Autodesk Fusion 360 part; units mm, degrees
(part 3 of 11)
  spline S32 degree 5 poles (-12.9257, -25.5744) (-12.9262, -25.5771) (-12.9273, -25.5825) (-12.9286, -25.5906) (-12.93, -25.6015) (-12.9313, -25.6152) (-12.9322, -25.629) (-12.9328, -25.6428) (-12.9334, -25.6566) (-12.9338, -25.6705) (-12.9341, -25.6844) (-12.9343, -25.6983) (-12.9344, -25.7122) (-12.9342, -25.7262) (-12.9339, -25.7401) (-12.9334, -25.7542) (-12.9328, -25.7682) (-12.932, -25.7822) (-12.9311, -25.7963) (-12.9302, -25.8104) (-12.9291, -25.8245) (-12.9279, -25.8386) (-12.9266, -25.8527) (-12.9252, -25.8669) (-12.9236, -25.8811) (-12.922, -25.8952) (-12.9202, -25.9094) (-12.9184, -25.9236) (-12.9164, -25.9378) (-12.9144, -25.9521) (-12.9122, -25.9663) (-12.91, -25.9805) (-12.9077, -25.9948) (-12.9052, -26.0091) (-12.9027, -26.0233) (-12.9001, -26.0376) (-12.8974, -26.0519) (-12.8946, -26.0662) (-12.8917, -26.0805) (-12.8887, -26.0948) (-12.8856, -26.1091) (-12.8825, -26.1235) (-12.8792, -26.1378) (-12.8759, -26.1521) (-12.8725, -26.1665) (-12.869, -26.1808) (-12.8655, -26.1952) (-12.8618, -26.2096) (-12.8581, -26.2239) (-12.8542, -26.2383) (-12.8503, -26.2527) (-12.8464, -26.267) (-12.8423, -26.2814) (-12.8382, -26.2958) (-12.834, -26.3102) (-12.8297, -26.3246) (-12.8253, -26.339) (-12.8209, -26.3534) (-12.8163, -26.3678) (-12.8117, -26.3822) (-12.8071, -26.3966) (-12.8023, -26.4109) (-12.7975, -26.4253) (-12.7926, -26.4397) (-12.7876, -26.4541) (-12.7826, -26.4685) (-12.7774, -26.4829) (-12.7722, -26.4973) (-12.767, -26.5117) (-12.7616, -26.5261) (-12.7562, -26.5405) (-12.7518, -26.5521) (-12.7485, -26.5607) (-12.7463, -26.5664) (-12.7452, -26.5693) knots 0 0 0 0 0 0 0.01428571 0.02857143 0.04285714 0.05714286 0.07142857 0.08571429 0.1 0.11428571 0.12857143 0.14285714 0.15714286 0.17142857 0.18571429 0.2 0.21428571 0.22857143 0.24285714 0.25714286 0.27142857 0.28571429 0.3 0.31428571 0.32857143 0.34285714 0.35714286 0.37142857 0.38571429 0.4 0.41428571 0.42857143 0.44285714 0.45714286 0.47142857 0.48571429 0.5 0.51428571 0.52857143 0.54285714 0.55714286 0.57142857 0.58571429 0.6 0.61428571 0.62857143 0.64285714 0.65714286 0.67142857 0.68571429 0.7 0.71428571 0.72857143 0.74285714 0.75714286 0.77142857 0.78571429 0.8 0.81428571 0.82857143 0.84285714 0.85714286 0.87142857 0.88571429 0.9 0.91428571 0.92857143 0.94285714 0.95714286 0.97142857 0.98571429 1 1 1 1 1 1
  arc A66 (-12.7452, -26.5693) -> (-12.3546, -26.6175) centre (-11.6741, -19.5) ccw
  spline S33 degree 5 poles (-12.3546, -26.6175) (-12.3528, -26.615) (-12.3493, -26.61) (-12.344, -26.6024) (-12.3369, -26.5923) (-12.3282, -26.5797) (-12.3195, -26.567) (-12.3109, -26.5543) (-12.3023, -26.5416) (-12.2939, -26.5289) (-12.2855, -26.5161) (-12.2771, -26.5034) (-12.2689, -26.4906) (-12.2607, -26.4778) (-12.2526, -26.465) (-12.2446, -26.4522) (-12.2366, -26.4393) (-12.2287, -26.4265) (-12.2209, -26.4136) (-12.2131, -26.4007) (-12.2055, -26.3878) (-12.1979, -26.3749) (-12.1904, -26.3619) (-12.183, -26.3489) (-12.1756, -26.336) (-12.1683, -26.323) (-12.1611, -26.31) (-12.154, -26.2969) (-12.147, -26.2839) (-12.14, -26.2708) (-12.1331, -26.2578) (-12.1263, -26.2447) (-12.1196, -26.2316) (-12.113, -26.2185) (-12.1065, -26.2053) (-12.1, -26.1922) (-12.0936, -26.179) (-12.0874, -26.1659) (-12.0812, -26.1527) (-12.0751, -26.1395) (-12.069, -26.1263) (-12.0631, -26.113) (-12.0573, -26.0998) (-12.0516, -26.0865) (-12.0459, -26.0733) (-12.0404, -26.06) (-12.0349, -26.0467) (-12.0296, -26.0334) (-12.0243, -26.02) (-12.0192, -26.0067) (-12.0141, -25.9933) (-12.0092, -25.98) (-12.0044, -25.9666) (-11.9997, -25.9532) (-11.9951, -25.9398) (-11.9906, -25.9264) (-11.9862, -25.913) (-11.982, -25.8995) (-11.9778, -25.8861) (-11.9738, -25.8726) (-11.9699, -25.8592) (-11.9662, -25.8457) (-11.9627, -25.8322) (-11.9593, -25.8186) (-11.9561, -25.8051) (-11.9531, -25.7916) (-11.9501, -25.778) (-11.9472, -25.7645) (-11.9445, -25.7509) (-11.942, -25.7373) (-11.9399, -25.7237) (-11.9387, -25.7128) (-11.938, -25.7046) (-11.9377, -25.6991) (-11.9376, -25.6964) knots -1 -1 -1 -1 -1 -1 -0.98571429 -0.97142857 -0.95714286 -0.94285714 -0.92857143 -0.91428571 -0.9 -0.88571429 -0.87142857 -0.85714286 -0.84285714 -0.82857143 -0.81428571 -0.8 -0.78571429 -0.77142857 -0.75714286 -0.74285714 -0.72857143 -0.71428571 -0.7 -0.68571429 -0.67142857 -0.65714286 -0.64285714 -0.62857143 -0.61428571 -0.6 -0.58571429 -0.57142857 -0.55714286 -0.54285714 -0.52857143 -0.51428571 -0.5 -0.48571429 -0.47142857 -0.45714286 -0.44285714 -0.42857143 -0.41428571 -0.4 -0.38571429 -0.37142857 -0.35714286 -0.34285714 -0.32857143 -0.31428571 -0.3 -0.28571429 -0.27142857 -0.25714286 -0.24285714 -0.22857143 -0.21428571 -0.2 -0.18571429 -0.17142857 -0.15714286 -0.14285714 -0.12857143 -0.11428571 -0.1 -0.08571429 -0.07142857 -0.05714286 -0.04285714 -0.02857143 -0.01428571 0 0 0 0 0 0
  line L33 (-11.9376, -25.6964) -> (-11.9345, -25.628)
  arc A67 (-11.6843, -25.3892) -> (-11.9345, -25.628) centre (-11.6847, -25.6392) ccw
  arc A68 (-11.6843, -25.3892) -> (-11.5691, -25.3883) centre (-11.6741, -19.5) ccw
  arc A69 (-11.3151, -25.623) -> (-11.5691, -25.3883) centre (-11.5646, -25.6382) ccw
  line L34 (-11.3151, -25.623) -> (-11.3109, -25.6913)
  spline S34 degree 5 poles (-11.3109, -25.6913) (-11.3107, -25.6941) (-11.3103, -25.6995) (-11.3095, -25.7077) (-11.3081, -25.7186) (-11.3057, -25.7322) (-11.303, -25.7457) (-11.3001, -25.7592) (-11.297, -25.7727) (-11.2938, -25.7862) (-11.2905, -25.7997) (-11.2871, -25.8132) (-11.2836, -25.8267) (-11.2798, -25.8401) (-11.2759, -25.8536) (-11.2718, -25.867) (-11.2676, -25.8804) (-11.2632, -25.8937) (-11.2587, -25.9071) (-11.2541, -25.9205) (-11.2494, -25.9338) (-11.2446, -25.9471) (-11.2397, -25.9604) (-11.2347, -25.9737) (-11.2295, -25.987) (-11.2243, -26.0003) (-11.2189, -26.0135) (-11.2134, -26.0268) (-11.2079, -26.04) (-11.2022, -26.0532) (-11.1964, -26.0664) (-11.1906, -26.0796) (-11.1846, -26.0927) (-11.1786, -26.1059) (-11.1725, -26.119) (-11.1662, -26.1321) (-11.1599, -26.1452) (-11.1535, -26.1583) (-11.147, -26.1714) (-11.1404, -26.1845) (-11.1338, -26.1975) (-11.127, -26.2105) (-11.1202, -26.2235) (-11.1133, -26.2365) (-11.1063, -26.2495) (-11.0992, -26.2625) (-11.092, -26.2754) (-11.0848, -26.2883) (-11.0774, -26.3012) (-11.07, -26.3141) (-11.0625, -26.327) (-11.055, -26.3399) (-11.0473, -26.3527) (-11.0396, -26.3655) (-11.0318, -26.3783) (-11.024, -26.3911) (-11.016, -26.4039) (-11.008, -26.4166) (-10.9999, -26.4294) (-10.9917, -26.4421) (-10.9835, -26.4548) (-10.9752, -26.4675) (-10.9668, -26.4801) (-10.9583, -26.4928) (-10.9498, -26.5054) (-10.9412, -26.518) (-10.9325, -26.5306) (-10.9238, -26.5431) (-10.915, -26.5557) (-10.9061, -26.5682) (-10.8971, -26.5807) (-10.8899, -26.5907) (-10.8845, -26.5982) (-10.8808, -26.6032) (-10.879, -26.6056) knots 0 0 0 0 0 0 0.01428571 0.02857143 0.04285714 0.05714286 0.07142857 0.08571429 0.1 0.11428571 0.12857143 0.14285714 0.15714286 0.17142857 0.18571429 0.2 0.21428571 0.22857143 0.24285714 0.25714286 0.27142857 0.28571429 0.3 0.31428571 0.32857143 0.34285714 0.35714286 0.37142857 0.38571429 0.4 0.41428571 0.42857143 0.44285714 0.45714286 0.47142857 0.48571429 0.5 0.51428571 0.52857143 0.54285714 0.55714286 0.57142857 0.58571429 0.6 0.61428571 0.62857143 0.64285714 0.65714286 0.67142857 0.68571429 0.7 0.71428571 0.72857143 0.74285714 0.75714286 0.77142857 0.78571429 0.8 0.81428571 0.82857143 0.84285714 0.85714286 0.87142857 0.88571429 0.9 0.91428571 0.92857143 0.94285714 0.95714286 0.97142857 0.98571429 1 1 1 1 1 1
  arc A70 (-10.879, -26.6056) -> (-10.4893, -26.5511) centre (-11.6741, -19.5) ccw
  spline S35 degree 5 poles (-10.4893, -26.5511) (-10.4882, -26.5482) (-10.4861, -26.5425) (-10.4829, -26.5338) (-10.4787, -26.5222) (-10.4735, -26.5077) (-10.4684, -26.4932) (-10.4634, -26.4787) (-10.4584, -26.4643) (-10.4535, -26.4498) (-10.4487, -26.4353) (-10.444, -26.4208) (-10.4393, -26.4063) (-10.4347, -26.3919) (-10.4302, -26.3774) (-10.4258, -26.3629) (-10.4214, -26.3485) (-10.4171, -26.334) (-10.4129, -26.3195) (-10.4087, -26.3051) (-10.4047, -26.2906) (-10.4007, -26.2762) (-10.3968, -26.2617) (-10.393, -26.2473) (-10.3892, -26.2328) (-10.3856, -26.2184) (-10.382, -26.204) (-10.3785, -26.1895) (-10.3751, -26.1751) (-10.3717, -26.1607) (-10.3685, -26.1463) (-10.3653, -26.1319) (-10.3622, -26.1175) (-10.3592, -26.1031) (-10.3563, -26.0888) (-10.3534, -26.0744) (-10.3507, -26.06) (-10.348, -26.0457) (-10.3455, -26.0313) (-10.343, -26.017) (-10.3406, -26.0027) (-10.3383, -25.9884) (-10.3361, -25.9741) (-10.334, -25.9598) (-10.332, -25.9455) (-10.3301, -25.9312) (-10.3282, -25.917) (-10.3265, -25.9027) (-10.3249, -25.8885) (-10.3234, -25.8743) (-10.3219, -25.8601) (-10.3206, -25.8459) (-10.3194, -25.8317) (-10.3184, -25.8176) (-10.3174, -25.8035) (-10.3165, -25.7893) (-10.3158, -25.7752) (-10.3151, -25.7612) (-10.3146, -25.7471) (-10.3142, -25.733) (-10.3139, -25.719) (-10.3139, -25.705) (-10.314, -25.6911) (-10.3142, -25.6771) (-10.3147, -25.6632) (-10.3152, -25.6494) (-10.3158, -25.6355) (-10.3166, -25.6217) (-10.3174, -25.6079) (-10.3186, -25.5941) (-10.32, -25.5805) (-10.3216, -25.5696) (-10.3231, -25.5615) (-10.3242, -25.5561) (-10.3248, -25.5534) knots -1 -1 -1 -1 -1 -1 -0.98571429 -0.97142857 -0.95714286 -0.94285714 -0.92857143 -0.91428571 -0.9 -0.88571429 -0.87142857 -0.85714286 -0.84285714 -0.82857143 -0.81428571 -0.8 -0.78571429 -0.77142857 -0.75714286 -0.74285714 -0.72857143 -0.71428571 -0.7 -0.68571429 -0.67142857 -0.65714286 -0.64285714 -0.62857143 -0.61428571 -0.6 -0.58571429 -0.57142857 -0.55714286 -0.54285714 -0.52857143 -0.51428571 -0.5 -0.48571429 -0.47142857 -0.45714286 -0.44285714 -0.42857143 -0.41428571 -0.4 -0.38571429 -0.37142857 -0.35714286 -0.34285714 -0.32857143 -0.31428571 -0.3 -0.28571429 -0.27142857 -0.25714286 -0.24285714 -0.22857143 -0.21428571 -0.2 -0.18571429 -0.17142857 -0.15714286 -0.14285714 -0.12857143 -0.11428571 -0.1 -0.08571429 -0.07142857 -0.05714286 -0.04285714 -0.02857143 -0.01428571 0 0 0 0 0 0
  line L35 (-10.3248, -25.5534) -> (-10.3396, -25.4865)
  arc A71 (-10.1597, -25.1912) -> (-10.3396, -25.4865) centre (-10.0954, -25.4327) ccw
  arc A72 (-10.1597, -25.1912) -> (-10.0486, -25.1604) centre (-11.6741, -19.5) ccw
  arc A73 (-9.7426, -25.3214) -> (-10.0486, -25.1604) centre (-9.9796, -25.4007) ccw
  line L36 (-9.7426, -25.3214) -> (-9.7208, -25.3863)
  spline S36 degree 5 poles (-9.7208, -25.3863) (-9.7199, -25.3889) (-9.7181, -25.3941) (-9.7152, -25.4018) (-9.711, -25.412) (-9.7053, -25.4245) (-9.6992, -25.4369) (-9.6928, -25.4492) (-9.6863, -25.4614) (-9.6798, -25.4736) (-9.6731, -25.4858) (-9.6663, -25.4979) (-9.6594, -25.51) (-9.6523, -25.5221) (-9.6451, -25.534) (-9.6376, -25.5459) (-9.6301, -25.5577) (-9.6224, -25.5695) (-9.6146, -25.5813) (-9.6067, -25.593) (-9.5987, -25.6047) (-9.5906, -25.6163) (-9.5824, -25.6279) (-9.5741, -25.6394) (-9.5657, -25.6509) (-9.5572, -25.6624) (-9.5486, -25.6738) (-9.5399, -25.6851) (-9.5311, -25.6965) (-9.5222, -25.7078) (-9.5132, -25.719) (-9.5042, -25.7302) (-9.495, -25.7414) (-9.4858, -25.7526) (-9.4764, -25.7637) (-9.467, -25.7747) (-9.4575, -25.7857) (-9.448, -25.7967) (-9.4383, -25.8077) (-9.4286, -25.8186) (-9.4187, -25.8294) (-9.4089, -25.8403) (-9.3989, -25.8511) (-9.3888, -25.8618) (-9.3787, -25.8725) (-9.3685, -25.8832) (-9.3582, -25.8939) (-9.3479, -25.9045) (-9.3375, -25.9151) (-9.327, -25.9256) (-9.3164, -25.9361) (-9.3058, -25.9465) (-9.2951, -25.957) (-9.2843, -25.9674) (-9.2735, -25.9777) (-9.2626, -25.988) (-9.2516, -25.9983) (-9.2405, -26.0085) (-9.2294, -26.0187) (-9.2182, -26.0289) (-9.207, -26.039) (-9.1957, -26.0491) (-9.1843, -26.0592) (-9.1729, -26.0692) (-9.1614, -26.0792) (-9.1498, -26.0891) (-9.1382, -26.0991) (-9.1265, -26.1089) (-9.1147, -26.1188) (-9.1029, -26.1286) (-9.091, -26.1383) (-9.0814, -26.1461) (-9.0742, -26.1519) (-9.0694, -26.1558) (-9.067, -26.1577) knots 0 0 0 0 0 0 0.01428571 0.02857143 0.04285714 0.05714286 0.07142857 0.08571429 0.1 0.11428571 0.12857143 0.14285714 0.15714286 0.17142857 0.18571429 0.2 0.21428571 0.22857143 0.24285714 0.25714286 0.27142857 0.28571429 0.3 0.31428571 0.32857143 0.34285714 0.35714286 0.37142857 0.38571429 0.4 0.41428571 0.42857143 0.44285714 0.45714286 0.47142857 0.48571429 0.5 0.51428571 0.52857143 0.54285714 0.55714286 0.57142857 0.58571429 0.6 0.61428571 0.62857143 0.64285714 0.65714286 0.67142857 0.68571429 0.7 0.71428571 0.72857143 0.74285714 0.75714286 0.77142857 0.78571429 0.8 0.81428571 0.82857143 0.84285714 0.85714286 0.87142857 0.88571429 0.9 0.91428571 0.92857143 0.94285714 0.95714286 0.97142857 0.98571429 1 1 1 1 1 1
  arc A74 (-9.067, -26.1577) -> (-8.7047, -26.0042) centre (-11.6741, -19.5) ccw
  spline S37 degree 5 poles (-8.7047, -26.0042) (-8.7044, -26.0011) (-8.7038, -25.995) (-8.703, -25.9858) (-8.702, -25.9735) (-8.7007, -25.9582) (-8.6995, -25.9429) (-8.6984, -25.9276) (-8.6974, -25.9123) (-8.6964, -25.8971) (-8.6955, -25.8818) (-8.6947, -25.8666) (-8.6939, -25.8514) (-8.6932, -25.8362) (-8.6926, -25.8211) (-8.692, -25.806) (-8.6916, -25.7909) (-8.6912, -25.7758) (-8.6908, -25.7607) (-8.6906, -25.7457) (-8.6904, -25.7307) (-8.6903, -25.7157) (-8.6903, -25.7007) (-8.6903, -25.6858) (-8.6904, -25.6709) (-8.6906, -25.656) (-8.6909, -25.6411) (-8.6912, -25.6263) (-8.6917, -25.6114) (-8.6922, -25.5967) (-8.6928, -25.5819) (-8.6934, -25.5672) (-8.6942, -25.5525) (-8.695, -25.5378) (-8.6959, -25.5232) (-8.6969, -25.5086) (-8.6979, -25.494) (-8.6991, -25.4794) (-8.7003, -25.4649) (-8.7016, -25.4504) (-8.703, -25.436) (-8.7045, -25.4215) (-8.7061, -25.4072) (-8.7077, -25.3928) (-8.7095, -25.3785) (-8.7113, -25.3642) (-8.7133, -25.35) (-8.7153, -25.3358) (-8.7174, -25.3216) (-8.7196, -25.3075) (-8.7219, -25.2934) (-8.7243, -25.2794) (-8.7268, -25.2654) (-8.7294, -25.2514) (-8.7322, -25.2375) (-8.735, -25.2237) (-8.7379, -25.2098) (-8.741, -25.1961) (-8.7441, -25.1824) (-8.7473, -25.1687) (-8.7507, -25.1551) (-8.7542, -25.1415) (-8.7579, -25.1281) (-8.7618, -25.1147) (-8.7658, -25.1014) (-8.7699, -25.0881) (-8.7741, -25.0749) (-8.7784, -25.0617) (-8.7828, -25.0486) (-8.7875, -25.0356) (-8.7924, -25.0228) (-8.7968, -25.0127) (-8.8003, -25.0053) (-8.8028, -25.0004) (-8.8041, -24.9979) knots -1 -1 -1 -1 -1 -1 -0.98571429 -0.97142857 -0.95714286 -0.94285714 -0.92857143 -0.91428571 -0.9 -0.88571429 -0.87142857 -0.85714286 -0.84285714 -0.82857143 -0.81428571 -0.8 -0.78571429 -0.77142857 -0.75714286 -0.74285714 -0.72857143 -0.71428571 -0.7 -0.68571429 -0.67142857 -0.65714286 -0.64285714 -0.62857143 -0.61428571 -0.6 -0.58571429 -0.57142857 -0.55714286 -0.54285714 -0.52857143 -0.51428571 -0.5 -0.48571429 -0.47142857 -0.45714286 -0.44285714 -0.42857143 -0.41428571 -0.4 -0.38571429 -0.37142857 -0.35714286 -0.34285714 -0.32857143 -0.31428571 -0.3 -0.28571429 -0.27142857 -0.25714286 -0.24285714 -0.22857143 -0.21428571 -0.2 -0.18571429 -0.17142857 -0.15714286 -0.14285714 -0.12857143 -0.11428571 -0.1 -0.08571429 -0.07142857 -0.05714286 -0.04285714 -0.02857143 -0.01428571 0 0 0 0 0 0
  line L37 (-8.8041, -24.9979) -> (-8.8356, -24.9371)
  arc A75 (-8.7383, -24.6053) -> (-8.8356, -24.9371) centre (-8.6137, -24.822) ccw
  arc A76 (-8.7383, -24.6053) -> (-8.639, -24.5468) centre (-11.6741, -19.5) ccw
  arc A77 (-8.3017, -24.6231) -> (-8.639, -24.5468) centre (-8.5102, -24.7611) ccw
  line L38 (-8.3017, -24.6231) -> (-8.2639, -24.6802)
  spline S38 degree 5 poles (-8.2639, -24.6802) (-8.2624, -24.6825) (-8.2593, -24.687) (-8.2545, -24.6938) (-8.2478, -24.7025) (-8.239, -24.713) (-8.2299, -24.7234) (-8.2206, -24.7336) (-8.2112, -24.7438) (-8.2016, -24.7539) (-8.1921, -24.7639) (-8.1824, -24.7739) (-8.1726, -24.7838) (-8.1626, -24.7936) (-8.1525, -24.8032) (-8.1422, -24.8128) (-8.1319, -24.8223) (-8.1214, -24.8317) (-8.1108, -24.841) (-8.1002, -24.8503) (-8.0894, -24.8595) (-8.0786, -24.8686) (-8.0677, -24.8777) (-8.0567, -24.8867) (-8.0456, -24.8956) (-8.0344, -24.9045) (-8.0231, -24.9133) (-8.0118, -24.922) (-8.0003, -24.9307) (-7.9888, -24.9393) (-7.9772, -24.9478) (-7.9656, -24.9563) (-7.9539, -24.9647) (-7.942, -24.9731) (-7.9302, -24.9814) (-7.9182, -24.9897) (-7.9062, -24.9978) (-7.8941, -25.006) (-7.8819, -25.0141) (-7.8697, -25.0221) (-7.8574, -25.03) (-7.8451, -25.0379) (-7.8326, -25.0458) (-7.8201, -25.0536) (-7.8076, -25.0613) (-7.795, -25.069) (-7.7823, -25.0766) (-7.7696, -25.0842) (-7.7568, -25.0917) (-7.7439, -25.0992) (-7.731, -25.1066) (-7.718, -25.1139) (-7.705, -25.1212) (-7.6919, -25.1285) (-7.6787, -25.1357) (-7.6655, -25.1428) (-7.6522, -25.1499) (-7.6389, -25.1569) (-7.6256, -25.1639) (-7.6121, -25.1708) (-7.5986, -25.1777) (-7.5851, -25.1845) (-7.5715, -25.1913) (-7.5579, -25.198) (-7.5442, -25.2047) (-7.5304, -25.2113) (-7.5166, -25.2178) (-7.5027, -25.2243) (-7.4888, -25.2308) (-7.4749, -25.2372) (-7.4609, -25.2436) (-7.4496, -25.2486) (-7.4412, -25.2524) (-7.4355, -25.2549) (-7.4327, -25.2561) knots 0 0 0 0 0 0 0.01428571 0.02857143 0.04285714 0.05714286 0.07142857 0.08571429 0.1 0.11428571 0.12857143 0.14285714 0.15714286 0.17142857 0.18571429 0.2 0.21428571 0.22857143 0.24285714 0.25714286 0.27142857 0.28571429 0.3 0.31428571 0.32857143 0.34285714 0.35714286 0.37142857 0.38571429 0.4 0.41428571 0.42857143 0.44285714 0.45714286 0.47142857 0.48571429 0.5 0.51428571 0.52857143 0.54285714 0.55714286 0.57142857 0.58571429 0.6 0.61428571 0.62857143 0.64285714 0.65714286 0.67142857 0.68571429 0.7 0.71428571 0.72857143 0.74285714 0.75714286 0.77142857 0.78571429 0.8 0.81428571 0.82857143 0.84285714 0.85714286 0.87142857 0.88571429 0.9 0.91428571 0.92857143 0.94285714 0.95714286 0.97142857 0.98571429 1 1 1 1 1 1
  arc A78 (-7.4327, -25.2561) -> (-7.1225, -25.014) centre (-11.6741, -19.5) ccw
  spline S39 degree 5 poles (-7.1225, -25.014) (-7.123, -25.011) (-7.124, -25.0049) (-7.1256, -24.9958) (-7.1278, -24.9837) (-7.1305, -24.9685) (-7.1333, -24.9534) (-7.1362, -24.9384) (-7.1392, -24.9234) (-7.1422, -24.9084) (-7.1452, -24.8934) (-7.1484, -24.8785) (-7.1516, -24.8637) (-7.1548, -24.8488) (-7.1582, -24.834) (-7.1615, -24.8193) (-7.165, -24.8046) (-7.1685, -24.7899) (-7.1721, -24.7753) (-7.1757, -24.7607) (-7.1795, -24.7461) (-7.1832, -24.7316) (-7.1871, -24.7171) (-7.191, -24.7027) (-7.195, -24.6883) (-7.199, -24.674) (-7.2031, -24.6597) (-7.2073, -24.6455) (-7.2115, -24.6313) (-7.2158, -24.6171) (-7.2202, -24.603) (-7.2247, -24.589) (-7.2292, -24.575) (-7.2338, -24.561) (-7.2384, -24.5471) (-7.2432, -24.5332) (-7.248, -24.5194) (-7.2529, -24.5057) (-7.2578, -24.492) (-7.2628, -24.4783) (-7.2679, -24.4647) (-7.2731, -24.4512) (-7.2783, -24.4377) (-7.2836, -24.4243) (-7.289, -24.4109) (-7.2945, -24.3976) (-7.3001, -24.3843) (-7.3057, -24.3711) (-7.3114, -24.358) (-7.3172, -24.3449) (-7.3231, -24.3319) (-7.329, -24.319) (-7.3351, -24.3061) (-7.3412, -24.2933) (-7.3474, -24.2806) (-7.3538, -24.2679) (-7.3602, -24.2553) (-7.3666, -24.2428) (-7.3732, -24.2304) (-7.3799, -24.218) (-7.3867, -24.2057) (-7.3936, -24.1936) (-7.4006, -24.1815) (-7.4078, -24.1696) (-7.4152, -24.1578) (-7.4226, -24.146) (-7.4301, -24.1344) (-7.4376, -24.1228) (-7.4453, -24.1112) (-7.4531, -24.0999) (-7.4612, -24.0888) (-7.4681, -24.0802) (-7.4734, -24.0739) (-7.477, -24.0698) (-7.4789, -24.0678) knots -1 -1 -1 -1 -1 -1 -0.98571429 -0.97142857 -0.95714286 -0.94285714 -0.92857143 -0.91428571 -0.9 -0.88571429 -0.87142857 -0.85714286 -0.84285714 -0.82857143 -0.81428571 -0.8 -0.78571429 -0.77142857 -0.75714286 -0.74285714 -0.72857143 -0.71428571 -0.7 -0.68571429 -0.67142857 -0.65714286 -0.64285714 -0.62857143 -0.61428571 -0.6 -0.58571429 -0.57142857 -0.55714286 -0.54285714 -0.52857143 -0.51428571 -0.5 -0.48571429 -0.47142857 -0.45714286 -0.44285714 -0.42857143 -0.41428571 -0.4 -0.38571429 -0.37142857 -0.35714286 -0.34285714 -0.32857143 -0.31428571 -0.3 -0.28571429 -0.27142857 -0.25714286 -0.24285714 -0.22857143 -0.21428571 -0.2 -0.18571429 -0.17142857 -0.15714286 -0.14285714 -0.12857143 -0.11428571 -0.1 -0.08571429 -0.07142857 -0.05714286 -0.04285714 -0.02857143 -0.01428571 0 0 0 0 0 0
  line L39 (-7.4789, -24.0678) -> (-7.5251, -24.0172)
  arc A79 (-7.517, -23.6715) -> (-7.5251, -24.0172) centre (-7.3406, -23.8486) ccw
  arc A80 (-7.517, -23.6715) -> (-7.4362, -23.5893) centre (-11.6741, -19.5) ccw
  arc A81 (-7.0906, -23.5757) -> (-7.4362, -23.5893) centre (-7.2563, -23.7629) ccw
  line L40 (-7.0906, -23.5757) -> (-7.0393, -23.6211)
  spline S40 degree 5 poles (-7.0393, -23.6211) (-7.0373, -23.6229) (-7.0331, -23.6265) (-7.0268, -23.6317) (-7.018, -23.6384) (-7.0068, -23.6463) (-6.9953, -23.654) (-6.9837, -23.6615) (-6.972, -23.6688) (-6.9602, -23.6761) (-6.9483, -23.6833) (-6.9364, -23.6905) (-6.9243, -23.6975) (-6.9122, -23.7043) (-6.8999, -23.7111) (-6.8875, -23.7177) (-6.8751, -23.7241) (-6.8625, -23.7305) (-6.8499, -23.7368) (-6.8372, -23.743) (-6.8244, -23.7491) (-6.8116, -23.7551) (-6.7987, -23.761) (-6.7858, -23.7669) (-6.7727, -23.7726) (-6.7596, -23.7783) (-6.7465, -23.7839) (-6.7332, -23.7894) (-6.72, -23.7948) (-6.7066, -23.8001) (-6.6932, -23.8054) (-6.6798, -23.8106) (-6.6662, -23.8157) (-6.6527, -23.8207) (-6.639, -23.8256) (-6.6254, -23.8305) (-6.6116, -23.8353) (-6.5979, -23.84) (-6.584, -23.8447) (-6.5701, -23.8492) (-6.5562, -23.8538) (-6.5422, -23.8582) (-6.5282, -23.8626) (-6.5141, -23.8668) (-6.5, -23.8711) (-6.4858, -23.8752) (-6.4716, -23.8793) (-6.4573, -23.8833) (-6.443, -23.8873) (-6.4287, -23.8911) (-6.4143, -23.895) (-6.3998, -23.8987) (-6.3853, -23.9024) (-6.3708, -23.906) (-6.3563, -23.9095) (-6.3416, -23.913) (-6.327, -23.9164) (-6.3123, -23.9198) (-6.2976, -23.923) (-6.2828, -23.9263) (-6.268, -23.9294) (-6.2532, -23.9325) (-6.2383, -23.9355) (-6.2234, -23.9385) (-6.2084, -23.9414) (-6.1934, -23.9442) (-6.1784, -23.947) (-6.1633, -23.9497) (-6.1482, -23.9523) (-6.1331, -23.9549) (-6.1179, -23.9574) (-6.1057, -23.9593) (-6.0966, -23.9608) (-6.0905, -23.9617) (-6.0874, -23.9622) knots 0 0 0 0 0 0 0.01428571 0.02857143 0.04285714 0.05714286 0.07142857 0.08571429 0.1 0.11428571 0.12857143 0.14285714 0.15714286 0.17142857 0.18571429 0.2 0.21428571 0.22857143 0.24285714 0.25714286 0.27142857 0.28571429 0.3 0.31428571 0.32857143 0.34285714 0.35714286 0.37142857 0.38571429 0.4 0.41428571 0.42857143 0.44285714 0.45714286 0.47142857 0.48571429 0.5 0.51428571 0.52857143 0.54285714 0.55714286 0.57142857 0.58571429 0.6 0.61428571 0.62857143 0.64285714 0.65714286 0.67142857 0.68571429 0.7 0.71428571 0.72857143 0.74285714 0.75714286 0.77142857 0.78571429 0.8 0.81428571 0.82857143 0.84285714 0.85714286 0.87142857 0.88571429 0.9 0.91428571 0.92857143 0.94285714 0.95714286 0.97142857 0.98571429 1 1 1 1 1 1
  arc A82 (-6.0874, -23.9622) -> (-5.8504, -23.6481) centre (-11.6741, -19.5) ccw
  spline S41 degree 5 poles (-5.8504, -23.6481) (-5.8517, -23.6453) (-5.8543, -23.6397) (-5.8582, -23.6313) (-5.8634, -23.6201) (-5.87, -23.6062) (-5.8766, -23.5924) (-5.8833, -23.5786) (-5.89, -23.5648) (-5.8968, -23.5511) (-5.9036, -23.5375) (-5.9105, -23.5239) (-5.9175, -23.5104) (-5.9245, -23.4969) (-5.9315, -23.4835) (-5.9386, -23.4701) (-5.9457, -23.4568) (-5.9529, -23.4435) (-5.9602, -23.4303) (-5.9675, -23.4171) (-5.9748, -23.4041) (-5.9822, -23.391) (-5.9897, -23.378) (-5.9972, -23.3651) (-6.0047, -23.3523) (-6.0124, -23.3395) (-6.02, -23.3267) (-6.0277, -23.3141) (-6.0355, -23.3014) (-6.0433, -23.2889) (-6.0512, -23.2764) (-6.0592, -23.264) (-6.0672, -23.2516) (-6.0752, -23.2393) (-6.0833, -23.2271) (-6.0915, -23.2149) (-6.0997, -23.2028) (-6.1079, -23.1908) (-6.1163, -23.1788) (-6.1246, -23.1669) (-6.1331, -23.1551) (-6.1416, -23.1434) (-6.1501, -23.1317) (-6.1588, -23.1201) (-6.1674, -23.1086) (-6.1762, -23.0972) (-6.185, -23.0858) (-6.1938, -23.0745) (-6.2027, -23.0633) (-6.2117, -23.0522) (-6.2207, -23.0411) (-6.2298, -23.0302) (-6.239, -23.0193) (-6.2483, -23.0085) (-6.2576, -22.9979) (-6.2669, -22.9873) (-6.2764, -22.9768) (-6.2859, -22.9664) (-6.2955, -22.956) (-6.3051, -22.9458) (-6.3148, -22.9357) (-6.3247, -22.9258) (-6.3346, -22.916) (-6.3446, -22.9063) (-6.3548, -22.8968) (-6.365, -22.8874) (-6.3752, -22.878) (-6.3855, -22.8687) (-6.3959, -22.8596) (-6.4064, -22.8507) (-6.4171, -22.842) (-6.4259, -22.8355) (-6.4327, -22.8308) (-6.4373, -22.8278) (-6.4396, -22.8263) knots -1 -1 -1 -1 -1 -1 -0.98571429 -0.97142857 -0.95714286 -0.94285714 -0.92857143 -0.91428571 -0.9 -0.88571429 -0.87142857 -0.85714286 -0.84285714 -0.82857143 -0.81428571 -0.8 -0.78571429 -0.77142857 -0.75714286 -0.74285714 -0.72857143 -0.71428571 -0.7 -0.68571429 -0.67142857 -0.65714286 -0.64285714 -0.62857143 -0.61428571 -0.6 -0.58571429 -0.57142857 -0.55714286 -0.54285714 -0.52857143 -0.51428571 -0.5 -0.48571429 -0.47142857 -0.45714286 -0.44285714 -0.42857143 -0.41428571 -0.4 -0.38571429 -0.37142857 -0.35714286 -0.34285714 -0.32857143 -0.31428571 -0.3 -0.28571429 -0.27142857 -0.25714286 -0.24285714 -0.22857143 -0.21428571 -0.2 -0.18571429 -0.17142857 -0.15714286 -0.14285714 -0.12857143 -0.11428571 -0.1 -0.08571429 -0.07142857 -0.05714286 -0.04285714 -0.02857143 -0.01428571 0 0 0 0 0 0
  line L41 (-6.4396, -22.8263) -> (-6.4973, -22.7894)
  arc A83 (-6.579, -22.4534) -> (-6.4973, -22.7894) centre (-6.3627, -22.5788) ccw
  arc A84 (-6.579, -22.4534) -> (-6.5222, -22.3531) centre (-11.6741, -19.5) ccw
  arc A85 (-6.192, -22.2505) -> (-6.5222, -22.3531) centre (-6.3035, -22.4742) ccw
  line L42 (-6.192, -22.2505) -> (-6.1307, -22.2811)
  spline S42 degree 5 poles (-6.1307, -22.2811) (-6.1282, -22.2823) (-6.1233, -22.2847) (-6.1158, -22.2881) (-6.1056, -22.2923) (-6.0927, -22.2971) (-6.0796, -22.3015) (-6.0665, -22.3057) (-6.0532, -22.3098) (-6.0399, -22.3137) (-6.0266, -22.3177) (-6.0132, -22.3215) (-5.9998, -22.3251) (-5.9863, -22.3286) (-5.9727, -22.3319) (-5.959, -22.3351) (-5.9453, -22.3381) (-5.9315, -22.341) (-5.9177, -22.3438) (-5.9038, -22.3465) (-5.8899, -22.3491) (-5.876, -22.3516) (-5.862, -22.354) (-5.848, -22.3563) (-5.8339, -22.3585) (-5.8198, -22.3606) (-5.8056, -22.3625) (-5.7914, -22.3644) (-5.7772, -22.3662) (-5.7629, -22.3679) (-5.7486, -22.3695) (-5.7343, -22.371) (-5.7199, -22.3725) (-5.7055, -22.3738) (-5.6911, -22.3751) (-5.6766, -22.3762) (-5.6621, -22.3773) (-5.6475, -22.3783) (-5.633, -22.3792) (-5.6184, -22.38) (-5.6038, -22.3808) (-5.5891, -22.3814) (-5.5744, -22.382) (-5.5597, -22.3825) (-5.545, -22.383) (-5.5302, -22.3833) (-5.5154, -22.3836) (-5.5006, -22.3838) (-5.4857, -22.3839) (-5.4709, -22.3839) (-5.456, -22.3838) (-5.4411, -22.3837) (-5.4261, -22.3835) (-5.4112, -22.3833) (-5.3962, -22.3829) (-5.3812, -22.3825) (-5.3661, -22.382) (-5.3511, -22.3814) (-5.336, -22.3808) (-5.3209, -22.3801) (-5.3058, -22.3793) (-5.2907, -22.3784) (-5.2755, -22.3775) (-5.2603, -22.3765) (-5.2451, -22.3754) (-5.2299, -22.3742) (-5.2147, -22.373) (-5.1994, -22.3717) (-5.1842, -22.3704) (-5.1689, -22.3689) (-5.1536, -22.3674) (-5.1413, -22.3662) (-5.1321, -22.3652) (-5.126, -22.3646) (-5.1229, -22.3642) knots 0 0 0 0 0 0 0.01428571 0.02857143 0.04285714 0.05714286 0.07142857 0.08571429 0.1 0.11428571 0.12857143 0.14285714 0.15714286 0.17142857 0.18571429 0.2 0.21428571 0.22857143 0.24285714 0.25714286 0.27142857 0.28571429 0.3 0.31428571 0.32857143 0.34285714 0.35714286 0.37142857 0.38571429 0.4 0.41428571 0.42857143 0.44285714 0.45714286 0.47142857 0.48571429 0.5 0.51428571 0.52857143 0.54285714 0.55714286 0.57142857 0.58571429 0.6 0.61428571 0.62857143 0.64285714 0.65714286 0.67142857 0.68571429 0.7 0.71428571 0.72857143 0.74285714 0.75714286 0.77142857 0.78571429 0.8 0.81428571 0.82857143 0.84285714 0.85714286 0.87142857 0.88571429 0.9 0.91428571 0.92857143 0.94285714 0.95714286 0.97142857 0.98571429 1 1 1 1 1 1
  arc A86 (-5.1229, -22.3642) -> (-4.9752, -21.9995) centre (-11.6741, -19.5) ccw
  spline S43 degree 5 poles (-4.9752, -21.9995) (-4.9772, -21.9971) (-4.9812, -21.9923) (-4.9871, -21.9852) (-4.995, -21.9758) (-5.005, -21.9641) (-5.015, -21.9524) (-5.025, -21.9408) (-5.0351, -21.9293) (-5.0452, -21.9178) (-5.0553, -21.9064) (-5.0655, -21.8951) (-5.0757, -21.8838) (-5.0859, -21.8726) (-5.0962, -21.8614) (-5.1065, -21.8503) (-5.1168, -21.8393) (-5.1272, -21.8284) (-5.1376, -21.8175) (-5.1481, -21.8067) (-5.1586, -21.7959) (-5.1691, -21.7853) (-5.1797, -21.7747) (-5.1903, -21.7641) (-5.2009, -21.7537) (-5.2116, -21.7433) (-5.2223, -21.7329) (-5.233, -21.7227) (-5.2438, -21.7125) (-5.2546, -21.7024) (-5.2654, -21.6924) (-5.2763, -21.6825) (-5.2872, -21.6726) (-5.2982, -21.6628) (-5.3092, -21.6531) (-5.3202, -21.6434) (-5.3313, -21.6339) (-5.3424, -21.6244) (-5.3535, -21.615) (-5.3647, -21.6057) (-5.3759, -21.5965) (-5.3871, -21.5873) (-5.3984, -21.5782) (-5.4097, -21.5693) (-5.4211, -21.5604) (-5.4325, -21.5516) (-5.4439, -21.5429) (-5.4554, -21.5343) (-5.4669, -21.5258) (-5.4785, -21.5173) (-5.49, -21.509) (-5.5017, -21.5008) (-5.5133, -21.4927) (-5.5251, -21.4847) (-5.5368, -21.4768) (-5.5486, -21.469) (-5.5605, -21.4613) (-5.5723, -21.4537) (-5.5842, -21.4462) (-5.5962, -21.4388) (-5.6082, -21.4315) (-5.6203, -21.4245) (-5.6324, -21.4176) (-5.6446, -21.4109) (-5.6569, -21.4043) (-5.6692, -21.3978) (-5.6815, -21.3914) (-5.6938, -21.3852) (-5.7062, -21.379) (-5.7187, -21.3731) (-5.7313, -21.3675) (-5.7415, -21.3635) (-5.7492, -21.3607) (-5.7545, -21.359) (-5.7571, -21.3582) knots -1 -1 -1 -1 -1 -1 -0.98571429 -0.97142857 -0.95714286 -0.94285714 -0.92857143 -0.91428571 -0.9 -0.88571429 -0.87142857 -0.85714286 -0.84285714 -0.82857143 -0.81428571 -0.8 -0.78571429 -0.77142857 -0.75714286 -0.74285714 -0.72857143 -0.71428571 -0.7 -0.68571429 -0.67142857 -0.65714286 -0.64285714 -0.62857143 -0.61428571 -0.6 -0.58571429 -0.57142857 -0.55714286 -0.54285714 -0.52857143 -0.51428571 -0.5 -0.48571429 -0.47142857 -0.45714286 -0.44285714 -0.42857143 -0.41428571 -0.4 -0.38571429 -0.37142857 -0.35714286 -0.34285714 -0.32857143 -0.31428571 -0.3 -0.28571429 -0.27142857 -0.25714286 -0.24285714 -0.22857143 -0.21428571 -0.2 -0.18571429 -0.17142857 -0.15714286 -0.14285714 -0.12857143 -0.11428571 -0.1 -0.08571429 -0.07142857 -0.05714286 -0.04285714 -0.02857143 -0.01428571 0 0 0 0 0 0
  line L43 (-5.7571, -21.3582) -> (-5.8224, -21.3375)
  arc A87 (-5.9882, -21.034) -> (-5.8224, -21.3375) centre (-5.7469, -21.0992) ccw
  arc A88 (-5.9882, -21.034) -> (-5.9593, -20.9225) centre (-11.6741, -19.5) ccw
  arc A89 (-5.6669, -20.7379) -> (-5.9593, -20.9225) centre (-5.7167, -20.9829) ccw
  line L44 (-5.6669, -20.7379) -> (-5.5998, -20.7515)
  spline S44 degree 5 poles (-5.5998, -20.7515) (-5.5971, -20.7521) (-5.5917, -20.7531) (-5.5835, -20.7545) (-5.5726, -20.7559) (-5.5589, -20.7572) (-5.5452, -20.7581) (-5.5314, -20.7587) (-5.5175, -20.7592) (-5.5037, -20.7596) (-5.4898, -20.76) (-5.4759, -20.7602) (-5.4619, -20.7602) (-5.448, -20.7601) (-5.434, -20.7598) (-5.42, -20.7593) (-5.4059, -20.7587) (-5.3919, -20.7579) (-5.3778, -20.757) (-5.3637, -20.756) (-5.3496, -20.755) (-5.3355, -20.7538) (-5.3214, -20.7525) (-5.3072, -20.751) (-5.2931, -20.7495) (-5.2789, -20.7479) (-5.2647, -20.7461) (-5.2505, -20.7443) (-5.2363, -20.7423) (-5.2221, -20.7402) (-5.2078, -20.7381) (-5.1936, -20.7359) (-5.1793, -20.7335) (-5.1651, -20.7311) (-5.1508, -20.7286) (-5.1365, -20.7259) (-5.1222, -20.7232) (-5.1079, -20.7204) (-5.0936, -20.7175) (-5.0793, -20.7146) (-5.065, -20.7115) (-5.0507, -20.7083) (-5.0363, -20.7051) (-5.022, -20.7018) (-5.0076, -20.6984) (-4.9933, -20.6949) (-4.9789, -20.6913) (-4.9646, -20.6877) (-4.9502, -20.6839) (-4.9358, -20.6801) (-4.9215, -20.6762) (-4.9071, -20.6722) (-4.8927, -20.6682) (-4.8783, -20.664) (-4.8639, -20.6598) (-4.8496, -20.6555) (-4.8352, -20.6512) (-4.8208, -20.6467) (-4.8064, -20.6422) (-4.792, -20.6376) (-4.7776, -20.6329) (-4.7632, -20.6282) (-4.7488, -20.6233) (-4.7344, -20.6184) (-4.72, -20.6135) (-4.7056, -20.6084) (-4.6912, -20.6033) (-4.6768, -20.5981) (-4.6624, -20.5928) (-4.648, -20.5875) (-4.6336, -20.5821) (-4.6221, -20.5777) (-4.6134, -20.5744) (-4.6077, -20.5722) (-4.6048, -20.571) knots 0 0 0 0 0 0 0.01428571 0.02857143 0.04285714 0.05714286 0.07142857 0.08571429 0.1 0.11428571 0.12857143 0.14285714 0.15714286 0.17142857 0.18571429 0.2 0.21428571 0.22857143 0.24285714 0.25714286 0.27142857 0.28571429 0.3 0.31428571 0.32857143 0.34285714 0.35714286 0.37142857 0.38571429 0.4 0.41428571 0.42857143 0.44285714 0.45714286 0.47142857 0.48571429 0.5 0.51428571 0.52857143 0.54285714 0.55714286 0.57142857 0.58571429 0.6 0.61428571 0.62857143 0.64285714 0.65714286 0.67142857 0.68571429 0.7 0.71428571 0.72857143 0.74285714 0.75714286 0.77142857 0.78571429 0.8 0.81428571 0.82857143 0.84285714 0.85714286 0.87142857 0.88571429 0.9 0.91428571 0.92857143 0.94285714 0.95714286 0.97142857 0.98571429 1 1 1 1 1 1
  arc A90 (-4.6048, -20.571) -> (-4.5566, -20.1805) centre (-11.6741, -19.5) ccw
  spline S45 degree 5 poles (-4.5566, -20.1805) (-4.5591, -20.1787) (-4.5642, -20.1751) (-4.5717, -20.1698) (-4.5818, -20.1628) (-4.5945, -20.154) (-4.6071, -20.1453) (-4.6198, -20.1367) (-4.6325, -20.1282) (-4.6453, -20.1197) (-4.658, -20.1113) (-4.6708, -20.103) (-4.6835, -20.0947) (-4.6963, -20.0866) (-4.7091, -20.0784) (-4.722, -20.0704) (-4.7348, -20.0624) (-4.7477, -20.0546) (-4.7605, -20.0467) (-4.7734, -20.039) (-4.7864, -20.0313) (-4.7993, -20.0238) (-4.8122, -20.0162) (-4.8252, -20.0088) (-4.8382, -20.0015) (-4.8512, -19.9942) (-4.8642, -19.987) (-4.8772, -19.9799) (-4.8902, -19.9728) (-4.9033, -19.9659) (-4.9164, -19.959) (-4.9294, -19.9522) (-4.9425, -19.9455) (-4.9557, -19.9389) (-4.9688, -19.9323) (-4.9819, -19.9259) (-4.9951, -19.9195) (-5.0083, -19.9132) (-5.0215, -19.907) (-5.0347, -19.9009) (-5.0479, -19.8949) (-5.0611, -19.889) (-5.0744, -19.8832) (-5.0876, -19.8774) (-5.1009, -19.8718) (-5.1142, -19.8662) (-5.1275, -19.8608) (-5.1408, -19.8554) (-5.1541, -19.8502) (-5.1674, -19.845) (-5.1808, -19.84) (-5.1942, -19.835) (-5.2075, -19.8302) (-5.2209, -19.8255) (-5.2343, -19.8209) (-5.2477, -19.8165) (-5.2612, -19.8121) (-5.2746, -19.8078) (-5.288, -19.8037) (-5.3015, -19.7996) (-5.315, -19.7958) (-5.3285, -19.792) (-5.342, -19.7885) (-5.3555, -19.7852) (-5.369, -19.782) (-5.3826, -19.7789) (-5.3961, -19.776) (-5.4097, -19.7731) (-5.4232, -19.7704) (-5.4368, -19.7679) (-5.4504, -19.7658) (-5.4613, -19.7645) (-5.4695, -19.7639) (-5.475, -19.7635) (-5.4778, -19.7634) knots -1 -1 -1 -1 -1 -1 -0.98571429 -0.97142857 -0.95714286 -0.94285714 -0.92857143 -0.91428571 -0.9 -0.88571429 -0.87142857 -0.85714286 -0.84285714 -0.82857143 -0.81428571 -0.8 -0.78571429 -0.77142857 -0.75714286 -0.74285714 -0.72857143 -0.71428571 -0.7 -0.68571429 -0.67142857 -0.65714286 -0.64285714 -0.62857143 -0.61428571 -0.6 -0.58571429 -0.57142857 -0.55714286 -0.54285714 -0.52857143 -0.51428571 -0.5 -0.48571429 -0.47142857 -0.45714286 -0.44285714 -0.42857143 -0.41428571 -0.4 -0.38571429 -0.37142857 -0.35714286 -0.34285714 -0.32857143 -0.31428571 -0.3 -0.28571429 -0.27142857 -0.25714286 -0.24285714 -0.22857143 -0.21428571 -0.2 -0.18571429 -0.17142857 -0.15714286 -0.14285714 -0.12857143 -0.11428571 -0.1 -0.08571429 -0.07142857 -0.05714286 -0.04285714 -0.02857143 -0.01428571 0 0 0 0 0 0
  line L45 (-5.4778, -19.7634) -> (-5.5462, -19.7603)
  arc A91 (-5.7849, -19.5102) -> (-5.5462, -19.7603) centre (-5.5349, -19.5106) ccw
  arc A92 (-5.7849, -19.5102) -> (-5.7859, -19.3949) centre (-11.6741, -19.5) ccw
  arc A93 (-5.5512, -19.1409) -> (-5.7859, -19.3949) centre (-5.5359, -19.3905) ccw
  line L46 (-5.5512, -19.1409) -> (-5.4828, -19.1367)
  spline S46 degree 5 poles (-5.4828, -19.1367) (-5.4801, -19.1366) (-5.4746, -19.1362) (-5.4664, -19.1354) (-5.4555, -19.1339) (-5.4419, -19.1316) (-5.4284, -19.1289) (-5.4149, -19.1259) (-5.4014, -19.1229) (-5.3879, -19.1197) (-5.3744, -19.1164) (-5.3609, -19.113) (-5.3474, -19.1094) (-5.334, -19.1057) (-5.3206, -19.1018) (-5.3072, -19.0977) (-5.2938, -19.0934) (-5.2804, -19.0891) (-5.267, -19.0846) (-5.2537, -19.08) (-5.2403, -19.0753) (-5.227, -19.0705) (-5.2137, -19.0656) (-5.2004, -19.0605) (-5.1871, -19.0554) (-5.1738, -19.0501) (-5.1606, -19.0448) (-5.1474, -19.0393) (-5.1341, -19.0337) (-5.1209, -19.0281) (-5.1077, -19.0223) (-5.0946, -19.0165) (-5.0814, -19.0105) (-5.0682, -19.0045) (-5.0551, -18.9983) (-5.042, -18.9921) (-5.0289, -18.9858) (-5.0158, -18.9794) (-5.0027, -18.9729) (-4.9897, -18.9663) (-4.9766, -18.9596) (-4.9636, -18.9529) (-4.9506, -18.9461) (-4.9376, -18.9391) (-4.9246, -18.9321) (-4.9117, -18.925) (-4.8987, -18.9179) (-4.8858, -18.9106) (-4.8729, -18.9033) (-4.86, -18.8959) (-4.8471, -18.8884) (-4.8343, -18.8808) (-4.8214, -18.8732) (-4.8086, -18.8655) (-4.7958, -18.8577) (-4.783, -18.8498) (-4.7703, -18.8419) (-4.7575, -18.8339) (-4.7448, -18.8258) (-4.7321, -18.8176) (-4.7194, -18.8094) (-4.7067, -18.801) (-4.694, -18.7927) (-4.6814, -18.7842) (-4.6688, -18.7757) (-4.6562, -18.7671) (-4.6436, -18.7584) (-4.631, -18.7496) (-4.6185, -18.7408) (-4.6059, -18.7319) (-4.5934, -18.723) (-4.5834, -18.7158) (-4.576, -18.7103) (-4.571, -18.7067) (-4.5685, -18.7049) knots 0 0 0 0 0 0 0.01428571 0.02857143 0.04285714 0.05714286 0.07142857 0.08571429 0.1 0.11428571 0.12857143 0.14285714 0.15714286 0.17142857 0.18571429 0.2 0.21428571 0.22857143 0.24285714 0.25714286 0.27142857 0.28571429 0.3 0.31428571 0.32857143 0.34285714 0.35714286 0.37142857 0.38571429 0.4 0.41428571 0.42857143 0.44285714 0.45714286 0.47142857 0.48571429 0.5 0.51428571 0.52857143 0.54285714 0.55714286 0.57142857 0.58571429 0.6 0.61428571 0.62857143 0.64285714 0.65714286 0.67142857 0.68571429 0.7 0.71428571 0.72857143 0.74285714 0.75714286 0.77142857 0.78571429 0.8 0.81428571 0.82857143 0.84285714 0.85714286 0.87142857 0.88571429 0.9 0.91428571 0.92857143 0.94285714 0.95714286 0.97142857 0.98571429 1 1 1 1 1 1
  arc A94 (-4.5685, -18.7049) -> (-4.623, -18.3152) centre (-11.6741, -19.5) ccw
  spline S47 degree 5 poles (-4.623, -18.3152) (-4.6259, -18.3141) (-4.6317, -18.3119) (-4.6404, -18.3088) (-4.652, -18.3046) (-4.6664, -18.2994) (-4.6809, -18.2943) (-4.6954, -18.2892) (-4.7099, -18.2843) (-4.7244, -18.2794) (-4.7388, -18.2746) (-4.7533, -18.2698) (-4.7678, -18.2652) (-4.7823, -18.2606) (-4.7967, -18.2561) (-4.8112, -18.2516) (-4.8257, -18.2473) (-4.8402, -18.243) (-4.8546, -18.2387) (-4.8691, -18.2346) (-4.8835, -18.2306) (-4.898, -18.2266) (-4.9124, -18.2227) (-4.9269, -18.2188) (-4.9413, -18.2151) (-4.9557, -18.2114) (-4.9702, -18.2078) (-4.9846, -18.2043) (-4.999, -18.2009) (-5.0134, -18.1976) (-5.0278, -18.1943) (-5.0422, -18.1911) (-5.0566, -18.1881) (-5.071, -18.185) (-5.0854, -18.1821) (-5.0997, -18.1793) (-5.1141, -18.1765) (-5.1285, -18.1739) (-5.1428, -18.1713) (-5.1571, -18.1688) (-5.1715, -18.1664) (-5.1858, -18.1642) (-5.2001, -18.1619) (-5.2144, -18.1598) (-5.2286, -18.1578) (-5.2429, -18.1559) (-5.2572, -18.1541) (-5.2714, -18.1524) (-5.2856, -18.1507) (-5.2999, -18.1492) (-5.3141, -18.1478) (-5.3282, -18.1465) (-5.3424, -18.1453) (-5.3566, -18.1442) (-5.3707, -18.1433) (-5.3848, -18.1424) (-5.3989, -18.1417) (-5.413, -18.141) (-5.4271, -18.1405) (-5.4411, -18.1401) (-5.4551, -18.1398) (-5.4691, -18.1397) (-5.4831, -18.1398) (-5.497, -18.1401) (-5.5109, -18.1405) (-5.5248, -18.1411) (-5.5386, -18.1417) (-5.5525, -18.1424) (-5.5663, -18.1433) (-5.58, -18.1444) (-5.5937, -18.1459) (-5.6046, -18.1475) (-5.6127, -18.149) (-5.618, -18.1501) (-5.6207, -18.1507) knots -1 -1 -1 -1 -1 -1 -0.98571429 -0.97142857 -0.95714286 -0.94285714 -0.92857143 -0.91428571 -0.9 -0.88571429 -0.87142857 -0.85714286 -0.84285714 -0.82857143 -0.81428571 -0.8 -0.78571429 -0.77142857 -0.75714286 -0.74285714 -0.72857143 -0.71428571 -0.7 -0.68571429 -0.67142857 -0.65714286 -0.64285714 -0.62857143 -0.61428571 -0.6 -0.58571429 -0.57142857 -0.55714286 -0.54285714 -0.52857143 -0.51428571 -0.5 -0.48571429 -0.47142857 -0.45714286 -0.44285714 -0.42857143 -0.41428571 -0.4 -0.38571429 -0.37142857 -0.35714286 -0.34285714 -0.32857143 -0.31428571 -0.3 -0.28571429 -0.27142857 -0.25714286 -0.24285714 -0.22857143 -0.21428571 -0.2 -0.18571429 -0.17142857 -0.15714286 -0.14285714 -0.12857143 -0.11428571 -0.1 -0.08571429 -0.07142857 -0.05714286 -0.04285714 -0.02857143 -0.01428571 0 0 0 0 0 0
  line L47 (-5.6207, -18.1507) -> (-5.6876, -18.1654)
  arc A95 (-5.983, -17.9856) -> (-5.6876, -18.1654) centre (-5.7414, -17.9213) ccw
  circle A96 centre (-11.6741, -19.5) radius 1.25
  line L48 (2.2523, -20.9132) -> (-9.7477, -20.9132)
  line L49 (-9.7477, -20.9132) -> (-9.7477, -18.9132)
  line L50 (-9.7477, -18.9132) -> (2.2523, -18.9132)
  line L51 (2.2523, -18.9132) -> (2.2523, -20.9132)
  line L52 (2.2523, -20.9132) -> (-9.7477, -18.9132) construction
  line L53 (-9.7477, -20.9132) -> (2.2523, -18.9132) construction
  arc A97 (-18.2736, -23.193) -> (-18.3043, -23.0819) centre (-23.9648, -24.7074) ccw construction
  arc A98 (-18.1434, -22.7758) -> (-18.3043, -23.0819) centre (-18.0641, -23.0129) ccw construction
  line L54 (-18.1434, -22.7758) -> (-18.0784, -22.7541) construction
  spline S48 degree 5 poles (-18.0784, -22.7541) (-18.0758, -22.7532) (-18.0706, -22.7514) (-18.0629, -22.7485) (-18.0528, -22.7443) (-18.0403, -22.7385) (-18.0279, -22.7324) (-18.0156, -22.7261) (-18.0034, -22.7196) (-17.9912, -22.713) (-17.979, -22.7064) (-17.9668, -22.6996) (-17.9547, -22.6927) (-17.9427, -22.6856) (-17.9308, -22.6783) (-17.9189, -22.6709) (-17.907, -22.6633) (-17.8952, -22.6556) (-17.8835, -22.6478) (-17.8718, -22.64) (-17.8601, -22.632) (-17.8485, -22.6239) (-17.8369, -22.6157) (-17.8254, -22.6074) (-17.8139, -22.599) (-17.8024, -22.5905) (-17.791, -22.5818) (-17.7796, -22.5731) (-17.7683, -22.5643) (-17.757, -22.5554) (-17.7457, -22.5465) (-17.7345, -22.5374) (-17.7234, -22.5283) (-17.7122, -22.519) (-17.7011, -22.5097) (-17.6901, -22.5003) (-17.679, -22.4908) (-17.6681, -22.4812) (-17.6571, -22.4716) (-17.6462, -22.4618) (-17.6353, -22.452) (-17.6245, -22.4421) (-17.6137, -22.4321) (-17.6029, -22.4221) (-17.5922, -22.412) (-17.5815, -22.4018) (-17.5709, -22.3915) (-17.5603, -22.3812) (-17.5497, -22.3707) (-17.5392, -22.3603) (-17.5287, -22.3497) (-17.5182, -22.3391) (-17.5078, -22.3284) (-17.4974, -22.3176) (-17.4871, -22.3067) (-17.4767, -22.2958) (-17.4665, -22.2848) (-17.4562, -22.2738) (-17.446, -22.2627) (-17.4359, -22.2515) (-17.4257, -22.2403) (-17.4156, -22.2289) (-17.4056, -22.2176) (-17.3955, -22.2061) (-17.3856, -22.1946) (-17.3756, -22.183) (-17.3657, -22.1714) (-17.3558, -22.1597) (-17.346, -22.148) (-17.3362, -22.1361) (-17.3264, -22.1242) (-17.3187, -22.1147) (-17.3128, -22.1075) (-17.309, -22.1027) (-17.307, -22.1003) knots 0 0 0 0 0 0 0.01428571 0.02857143 0.04285714 0.05714286 0.07142857 0.08571429 0.1 0.11428571 0.12857143 0.14285714 0.15714286 0.17142857 0.18571429 0.2 0.21428571 0.22857143 0.24285714 0.25714286 0.27142857 0.28571429 0.3 0.31428571 0.32857143 0.34285714 0.35714286 0.37142857 0.38571429 0.4 0.41428571 0.42857143 0.44285714 0.45714286 0.47142857 0.48571429 0.5 0.51428571 0.52857143 0.54285714 0.55714286 0.57142857 0.58571429 0.6 0.61428571 0.62857143 0.64285714 0.65714286 0.67142857 0.68571429 0.7 0.71428571 0.72857143 0.74285714 0.75714286 0.77142857 0.78571429 0.8 0.81428571 0.82857143 0.84285714 0.85714286 0.87142857 0.88571429 0.9 0.91428571 0.92857143 0.94285714 0.95714286 0.97142857 0.98571429 1 1 1 1 1 1 construction
  arc A99 (-17.307, -22.1003) -> (-17.4605, -21.738) centre (-23.9648, -24.7074) ccw construction
  spline S49 degree 5 poles (-17.4605, -21.738) (-17.4636, -21.7377) (-17.4698, -21.7371) (-17.479, -21.7363) (-17.4913, -21.7352) (-17.5066, -21.734) (-17.5219, -21.7328) (-17.5372, -21.7317) (-17.5525, -21.7306) (-17.5677, -21.7296) (-17.5829, -21.7287) (-17.5982, -21.7279) (-17.6134, -21.7272) (-17.6285, -21.7265) (-17.6437, -21.7258) (-17.6588, -21.7253) (-17.6739, -21.7248) (-17.689, -21.7244) (-17.704, -21.7241) (-17.7191, -21.7238) (-17.7341, -21.7237) (-17.7491, -21.7236) (-17.7641, -21.7235) (-17.779, -21.7236) (-17.7939, -21.7237) (-17.8088, -21.7239) (-17.8237, -21.7242) (-17.8385, -21.7245) (-17.8533, -21.7249) (-17.8681, -21.7254) (-17.8829, -21.726) (-17.8976, -21.7267) (-17.9123, -21.7274) (-17.927, -21.7282) (-17.9416, -21.7291) (-17.9562, -21.7301) (-17.9708, -21.7312) (-17.9853, -21.7323) (-17.9999, -21.7336) (-18.0144, -21.7349) (-18.0288, -21.7363) (-18.0432, -21.7378) (-18.0576, -21.7393) (-18.072, -21.741) (-18.0863, -21.7427) (-18.1006, -21.7446) (-18.1148, -21.7465) (-18.129, -21.7485) (-18.1432, -21.7506) (-18.1573, -21.7528) (-18.1714, -21.7552) (-18.1854, -21.7576) (-18.1994, -21.7601) (-18.2133, -21.7627) (-18.2273, -21.7654) (-18.2411, -21.7683) (-18.2549, -21.7712) (-18.2687, -21.7742) (-18.2824, -21.7773) (-18.2961, -21.7806) (-18.3097, -21.7839) (-18.3232, -21.7875) (-18.3367, -21.7912) (-18.3501, -21.7951) (-18.3634, -21.7991) (-18.3766, -21.8032) (-18.3899, -21.8074) (-18.403, -21.8117) (-18.4161, -21.8161) (-18.4291, -21.8207) (-18.442, -21.8257) (-18.4521, -21.8301) (-18.4595, -21.8336) (-18.4644, -21.8361) (-18.4668, -21.8373) knots -1 -1 -1 -1 -1 -1 -0.98571429 -0.97142857 -0.95714286 -0.94285714 -0.92857143 -0.91428571 -0.9 -0.88571429 -0.87142857 -0.85714286 -0.84285714 -0.82857143 -0.81428571 -0.8 -0.78571429 -0.77142857 -0.75714286 -0.74285714 -0.72857143 -0.71428571 -0.7 -0.68571429 -0.67142857 -0.65714286 -0.64285714 -0.62857143 -0.61428571 -0.6 -0.58571429 -0.57142857 -0.55714286 -0.54285714 -0.52857143 -0.51428571 -0.5 -0.48571429 -0.47142857 -0.45714286 -0.44285714 -0.42857143 -0.41428571 -0.4 -0.38571429 -0.37142857 -0.35714286 -0.34285714 -0.32857143 -0.31428571 -0.3 -0.28571429 -0.27142857 -0.25714286 -0.24285714 -0.22857143 -0.21428571 -0.2 -0.18571429 -0.17142857 -0.15714286 -0.14285714 -0.12857143 -0.11428571 -0.1 -0.08571429 -0.07142857 -0.05714286 -0.04285714 -0.02857143 -0.01428571 0 0 0 0 0 0 construction
  line L55 (-18.4668, -21.8373) -> (-18.5276, -21.8689) construction
  arc A100 (-18.8595, -21.7716) -> (-18.5276, -21.8689) centre (-18.6428, -21.647) ccw construction
  arc A101 (-18.8595, -21.7716) -> (-18.9179, -21.6723) centre (-23.9648, -24.7074) ccw construction
  arc A102 (-18.8417, -21.3349) -> (-18.9179, -21.6723) centre (-18.7037, -21.5434) ccw construction
  line L56 (-18.8417, -21.3349) -> (-18.7846, -21.2971) construction
  spline S50 degree 5 poles (-18.7846, -21.2971) (-18.7823, -21.2956) (-18.7777, -21.2925) (-18.771, -21.2877) (-18.7623, -21.281) (-18.7517, -21.2723) (-18.7414, -21.2631) (-18.7311, -21.2538) (-18.721, -21.2444) (-18.7109, -21.2349) (-18.7008, -21.2253) (-18.6909, -21.2156) (-18.681, -21.2058) (-18.6712, -21.1959) (-18.6615, -21.1857) (-18.652, -21.1755) (-18.6425, -21.1651) (-18.6331, -21.1546) (-18.6238, -21.1441) (-18.6145, -21.1334) (-18.6053, -21.1227) (-18.5961, -21.1119) (-18.5871, -21.1009) (-18.5781, -21.0899) (-18.5691, -21.0788) (-18.5603, -21.0677) (-18.5515, -21.0564) (-18.5428, -21.045) (-18.5341, -21.0336) (-18.5255, -21.0221) (-18.5169, -21.0105) (-18.5085, -20.9988) (-18.5, -20.9871) (-18.4917, -20.9753) (-18.4834, -20.9634) (-18.4751, -20.9515) (-18.4669, -20.9395) (-18.4588, -20.9274) (-18.4507, -20.9152) (-18.4427, -20.903) (-18.4347, -20.8907) (-18.4268, -20.8783) (-18.419, -20.8659) (-18.4112, -20.8534) (-18.4035, -20.8409) (-18.3958, -20.8282) (-18.3882, -20.8156) (-18.3806, -20.8028) (-18.3731, -20.79) (-18.3656, -20.7772) (-18.3582, -20.7642) (-18.3509, -20.7513) (-18.3436, -20.7382) (-18.3363, -20.7251) (-18.3291, -20.712) (-18.322, -20.6988) (-18.3149, -20.6855) (-18.3079, -20.6722) (-18.3009, -20.6588) (-18.294, -20.6454) (-18.2871, -20.6319) (-18.2803, -20.6184) (-18.2735, -20.6048) (-18.2668, -20.5911) (-18.2601, -20.5774) (-18.2535, -20.5637) (-18.2469, -20.5499) (-18.2404, -20.536) (-18.234, -20.5221) (-18.2276, -20.5081) (-18.2212, -20.4941) (-18.2162, -20.4829) (-18.2124, -20.4744) (-18.2099, -20.4688) (-18.2087, -20.466) knots 0 0 0 0 0 0 0.01428571 0.02857143 0.04285714 0.05714286 0.07142857 0.08571429 0.1 0.11428571 0.12857143 0.14285714 0.15714286 0.17142857 0.18571429 0.2 0.21428571 0.22857143 0.24285714 0.25714286 0.27142857 0.28571429 0.3 0.31428571 0.32857143 0.34285714 0.35714286 0.37142857 0.38571429 0.4 0.41428571 0.42857143 0.44285714 0.45714286 0.47142857 0.48571429 0.5 0.51428571 0.52857143 0.54285714 0.55714286 0.57142857 0.58571429 0.6 0.61428571 0.62857143 0.64285714 0.65714286 0.67142857 0.68571429 0.7 0.71428571 0.72857143 0.74285714 0.75714286 0.77142857 0.78571429 0.8 0.81428571 0.82857143 0.84285714 0.85714286 0.87142857 0.88571429 0.9 0.91428571 0.92857143 0.94285714 0.95714286 0.97142857 0.98571429 1 1 1 1 1 1 construction
  arc A103 (-18.2087, -20.466) -> (-18.4507, -20.1557) centre (-23.9648, -24.7074) ccw construction